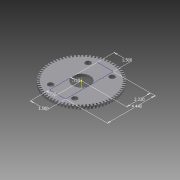
# Autodesk Inventor part: Gear
Saved by Autodesk Inventor 2015 (Build 190159000, 159)
## iProperties
Created: 2015-03-26
Part Number: Gear
Material: Generic
Document SubType Name: Modeling
Designer: WASHHSST
Density: 1 g/cm^3
Appearance: Default
Author: WASHHSST
Autodesk Inventor part; units mm, degrees
ref_plane "YZ Plane" through (0, 0, 0) normal (1, 0, 0) x (0, 1, 0)
ref_plane "XZ Plane" through (0, 0, 0) normal (0, 1, 0) x (-1, 0, 0)
ref_plane "XY Plane" through (0, 0, 0) normal (0, 0, 1) x (1, 0, 0)
sketch "Sketch1" plane through (0, 0, 0) normal (0, 1, 0) x (-1, 0, 0)
  circle A0 centre (0, 0) radius 74.676
  dimension "d0" = 149.352
  constraints: 1 centre point, 1 coincident
  measures "d0" diameter of A0
extrude "Extrusion1" add sketch "Sketch1" along normal blind 6.35
sketch "Sketch2" plane through (0, 6.35, 0) normal (0, 1, 0) x (1, 0, 0)
  point P0 (0, 0)
sketch "Sketch3" plane through (0, 6.35, 0) normal (0, 1, 0) x (1, 0, 0)
  arc A0 (0, 69.342) -> (-3.0247, 69.276) centre (0, 0) ccw
  circle A1 centre (0, 0) radius 74.676 projected
  line L0 (0, 69.342) -> (0, 74.676)
  line L1 (-3.0247, 69.276) -> (-3.2573, 74.6049)
  dimension "d3" = 138.684
  dimension "d4" = 2.5
  dimension "d6" = 5.334
  dimension "d7" = 5.3289
  constraints: 4 end point, 4 point on circle, 1 centre point, 1 coincident, 1 vertical
  measures "d3" diameter of A0
  measures "d4" angle of L0 L1
  measures "d6" distance of L0.end L0.start
  measures "d7" vertical distance of L1.start L1.end
extrude "Extrusion2" cut sketch "Sketch3" against normal blind 6.35 contours A0 L1 A1 L0 picked at (-0.362, 72.8954)
pattern_circular "Circular Pattern1" count 72 over 360 about axis through (0, -10, 0) along (0, 1, 0) of "Extrusion2"
sketch "Sketch4" plane through (0, 6.35, 0) normal (0, 1, 0) x (1, 0, 0)
  circle A0 centre (28.448, 44.196) radius 6.35
  circle A1 centre (28.448, -44.196) radius 6.35
  line L0 (19.05, 0) -> (19.05, 94.3603) construction
  line L1 (-19.05, 0) -> (-19.05, 94.3603) construction
  line L2 (28.448, 44.196) -> (28.448, -44.196) construction
  circle A2 centre (-28.448, 44.196) radius 6.35
  circle A3 centre (-28.448, -44.196) radius 6.35
  line L3 (-28.448, 94.3603) -> (-28.448, -90.76) construction
  line L4 (28.448, -44.196) -> (-81.305, -44.196) construction
  line L5 (28.448, 44.196) -> (-81.305, 44.196) construction
  point P0 (0, 0)
  point P1 (0, -74.676)
  point P2 (0, 74.676)
  dimension "d13" = 12.7
  dimension "d14" = 12.7
  dimension "d18" = 19.05
  dimension "d19" = 38.1
  dimension "d20" = 9.398
  dimension "d21" = 88.392
  dimension "d24" = 44.196
  dimension "d25" = 12.7
  dimension "d26" = 12.7
  dimension "d27" = 56.896
  constraints: 12 end point, 4 centre point, 4 point on line, 3 vertical, 2 horizontal, 1 coincident, 1 parallel
  measures "d13" diameter of A0
  measures "d14" diameter of A1
  measures "d18" distance from line of point (0, 0) L0
  measures "d19" distance between parallel lines of L0 L1
  measures "d20" distance from line of L0 L2.start
  measures "d21" distance of L2.start A1.centre
  measures "d24" vertical distance of L2.start point (0, 0)
  measures "d25" diameter of A2
  measures "d26" diameter of A3
  measures "d27" distance from line of L2.start L3
extrude "Extrusion3" cut sketch "Sketch4" against normal blind 6.35
sketch "Sketch5" plane through (0, 6.35, 0) normal (0, 1, 0) x (1, 0, 0)
  point P0 (0, 0)
sketch "Sketch6" plane through (0, 6.35, 0) normal (0, 1, 0) x (1, 0, 0)
  circle A0 centre (0, 0) radius 20.32
  dimension "d30" = 40.64
  constraints: 1 centre point, 1 coincident
  measures "d30" diameter of A0
extrude "Extrusion4" cut sketch "Sketch6" against normal blind 25.4
sketch "Sketch7" plane through (0, 6.35, 0) normal (0, 1, 0) x (1, 0, 0)
  line L0 (-19.05, -56.388) -> (19.05, -56.388) construction
  line L1 (-19.05, 56.388) -> (19.05, 56.388) construction
  line L2 (-19.05, -56.388) -> (-19.05, 56.388) construction
  line L3 (19.05, -56.388) -> (19.05, 56.388) construction
  point P0 (0, 0)
  dimension "d33" = 112.776
  dimension "d34" = 56.388
  dimension "d35" = 38.1
  dimension "d36" = 38.1
  dimension "d37" = 19.05
  dimension "d38" = 19.05
  constraints: 8 end point, 2 horizontal
  measures "d33" distance between parallel lines of L1 L0
  measures "d34" distance from line of L1 point (0, 0)
  measures "d35" distance of L1.end L1.start
  measures "d36" distance of L0.end L0.start
  measures "d37" horizontal distance of L1.start point (0, 0)
  measures "d38" horizontal distance of L0.start point (0, 0)
body "Solid1"
